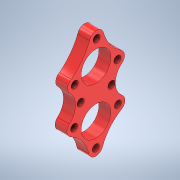
# Autodesk Inventor part: hw6
Saved by Autodesk Inventor 2021 (Build 250183000, 183)
## iProperties
Created: 2022-04-30
Part Number: hw6
Material: Generic
Document SubType Name: Modeling
Designer: authe
Density: 1 g/cm^3
Appearance: Light Red
Author: authe
Autodesk Inventor part; units mm, degrees
ref_plane "YZ Plane" through (0, 0, 0) normal (1, 0, 0) x (0, 1, 0)
ref_plane "XZ Plane" through (0, 0, 0) normal (0, 1, 0) x (-1, 0, 0)
ref_plane "XY Plane" through (0, 0, 0) normal (0, 0, 1) x (1, 0, 0)
sketch "Sketch2" plane through (0, 0, 0) normal (1, 0, 0) x (0, 1, 0)
  circle A0 centre (0, 0) radius 12.5
  line L0 (0, 0) -> (40, 0)
  circle A1 centre (40, 0) radius 12.5
  arc A2 (61.4867, -6.219) -> (61.2036, 5.4037) centre (59.8596, -0.4438) ccw
  circle A3 centre (59.8596, -0.4438) radius 3
  arc A4 (8.9245, 22.4355) -> (-0.904, 21.2616) centre (4.4125, 18.4805) ccw
  arc A5 (-2.1636, -21.4445) -> (7.7329, -22.0405) centre (2.9878, -18.3684) ccw
  arc A6 (31.2492, -21.7764) -> (40.9283, -21.2885) centre (35.9106, -17.9987) ccw
  arc A7 (40.7702, 20.8389) -> (36.9681, 12.1267) centre (35.5128, 17.9476) ccw
  line L1 (20, 0) -> (20, -13)
  line L2 (20, 0) -> (20, 13)
  arc A8 (-18.8462, 6.1399) -> (-21.6016, -5.4642) centre (-19.5799, 0.1849) ccw
  circle A9 centre (4.4125, 18.4805) radius 3
  circle A10 centre (2.9878, -18.3684) radius 3
  circle A11 centre (35.9106, -17.9987) radius 3
  circle A12 centre (35.5128, 17.9476) radius 3
  circle A13 centre (-19.5799, 0.1849) radius 3
  circle A14 centre (20, -13) radius 3
  circle A15 centre (20, 13) radius 3
  arc A16 (8.9245, 22.4355) -> (31.139, 22.0548) centre (20.2045, 32.323) ccw
  arc A17 (31.2492, -21.7764) -> (7.7329, -22.0405) centre (19.5956, -31.2207) ccw
  arc A18 (-2.1636, -21.4445) -> (-21.6016, -5.4642) centre (-34.1581, -40.5495) ccw
  arc A19 (-20.855, 6.0479) -> (-0.904, 21.2616) centre (-27.1495, 34.9909) ccw
  arc A20 (61.4867, -6.219) -> (40.9283, -21.2885) centre (71.3527, -41.2366) ccw
  arc A21 (7.2664, 17.5556) -> (-1.5702, 18.935) centre (0, 0) ccw
  arc A22 (40.7702, 20.8389) -> (61.2036, 5.4037) centre (79.072, 50.3008) ccw
  point P0 (-18.7745, -6.6085)
  point P1 (-17.6848, 6.9242)
  dimension "d4" = 25
  dimension "d22" = 6
  dimension "d1" = 25
  dimension "d3" = 40
  dimension "d6" = 12
  dimension "d7" = 6
  dimension "d12" = 12
  dimension "d13" = 12
  dimension "d15" = 12
  dimension "d16" = 12
  dimension "d17" = 13
  dimension "d18" = 13
  dimension "d21" = 12
  dimension "d23" = 6
  dimension "d24" = 6
  dimension "d25" = 6
  dimension "d26" = 6
  dimension "d27" = 6
  dimension "d28" = 6
  dimension "d29" = 15
  dimension "d30" = 15
  dimension "d31" = 37.2645
  dimension "d34" = 36.3809
  constraints: 32 point on circle, 21 centre point, 12 coincident, 10 tangent, 6 end point, 2 perpendicular, 1 horizontal, 1 midpoint, 7 other
  measures "d1" diameter of A0
  measures "d3" distance of L0.start L0.end
  measures "d6" diameter of A2
  measures "d7" diameter of A3
  measures "d12" diameter of A4
  measures "d13" diameter of A5
  measures "d15" diameter of A6
  measures "d16" diameter of A7
  measures "d17" distance of L1.start L1.end
  measures "d18" distance of L1.start L2.end
  measures "d21" diameter of A8
  measures "d23" diameter of A10
  measures "d24" diameter of A11
  measures "d25" diameter of A12
  measures "d26" diameter of A13
  measures "d27" diameter of A14
  measures "d28" diameter of A15
  measures "d29" radius of A16
  measures "d30" radius of A17
  measures "d31" radius of A18
  measures "d34" radius of A20
extrude "Extrusion1" add sketch "Sketch2" along normal mid plane 10
body "Solid1"
